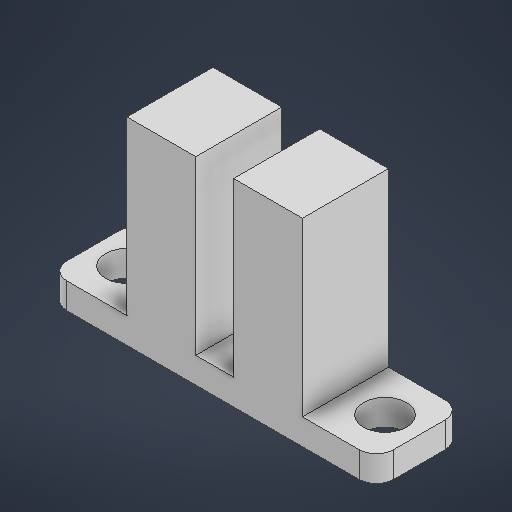
# Autodesk Inventor part: uchytka
Saved by Autodesk Inventor 2026.1 (Build 301233000, 233)
## iProperties
Created: 2026-01-08
Part Number: uchytka
Material: Všeobecné
Document SubType Name: Modeling
Designer: bubli
Density: 1 g/cm^3
Appearance: Výchozí
Author: bubli
Autodesk Inventor part; units mm, degrees
ref_plane "YZ Plane" through (0, 0, 0) normal (1, 0, 0) x (0, 1, 0)
ref_plane "XZ Plane" through (0, 0, 0) normal (0, 1, 0) x (-1, 0, 0)
ref_plane "XY Plane" through (0, 0, 0) normal (0, 0, 1) x (1, 0, 0)
sketch "Náčrt1" plane through (0, 0, 0) normal (0, 0, 1) x (1, 0, 0)
  line L0 (-6.3446, 3.6092) -> (27.6554, 3.6092)
  line L1 (29.6554, 1.6092) -> (29.6554, -4.3908)
  line L2 (27.6554, -6.3908) -> (-6.3446, -6.3908)
  line L3 (-8.3446, -4.3908) -> (-8.3446, 1.6092)
  circle A0 centre (-4.3446, -1.3908) radius 2.5
  circle A1 centre (25.6554, -1.3908) radius 2.5
  arc A2 (-6.3446, 3.6092) -> (-8.3446, 1.6092) centre (-6.3446, 1.6092) ccw
  arc A3 (29.6554, 1.6092) -> (27.6554, 3.6092) centre (27.6554, 1.6092) ccw
  arc A4 (27.6554, -6.3908) -> (29.6554, -4.3908) centre (27.6554, -4.3908) ccw
  arc A5 (-8.3446, -4.3908) -> (-6.3446, -6.3908) centre (-6.3446, -4.3908) ccw
  point P0 (0, 0)
  point P1 (-8.3446, 3.6092)
  point P2 (29.6554, 3.6092)
  point P3 (-8.3446, -6.3908)
  dimension "d0" = 38
  dimension "d1" = 10
  dimension "d2" = 5
  dimension "d3" = 5
  dimension "d4" = 5
  dimension "d5" = 5
  dimension "d6" = 4
  dimension "d7" = 4
  dimension "d8" = 2
  constraints: 8 end point, 8 point on circle, 8 tangent, 6 centre point, 6 point on line, 3 equal radius, 2 parallel, 1 horizontal, 1 perpendicular
  measures "d0" distance of point (-8.345, 3.609) point (29.655, 3.609)
  measures "d1" distance of point (-8.345, -6.391) point (-8.345, 3.609)
  measures "d2" diameter of A0
  measures "d3" diameter of A1
  measures "d4" distance from line of L0 A0.centre
  measures "d5" distance from line of L0 A1.centre
  measures "d6" distance from line of L3 A0.centre
  measures "d7" distance from line of L1 A1.centre
  measures "d8" radius of A2
extrude "Vysunutí1" add sketch "Náčrt1" along normal blind 3
sketch "Náčrt2" plane through (0, 0, 3) normal (0, 0, 1) x (1, 0, 0)
  line L0 (0.6554, 3.6092) -> (8.6554, 3.6092)
  line L1 (8.6554, 3.6092) -> (8.6554, -6.3908)
  line L2 (8.6554, -6.3908) -> (0.6554, -6.3908)
  line L3 (0.6554, -6.3908) -> (0.6554, 3.6092)
  line L4 (13.0554, 3.6092) -> (21.0554, 3.6092)
  line L5 (21.0554, 3.6092) -> (21.0554, -6.3908)
  line L6 (21.0554, -6.3908) -> (13.0554, -6.3908)
  line L7 (13.0554, -6.3908) -> (13.0554, 3.6092)
  line L8 (-8.3446, 1.6092) -> (-8.3446, -4.3908) projected
  line L9 (-6.3446, -6.3908) -> (27.6554, -6.3908) projected
  line L10 (27.6554, 3.6092) -> (-6.3446, 3.6092) projected
  point P0 (0, 0)
  point P1 (4.6554, -6.3908)
  dimension "d11" = 4.4
  dimension "d12" = 8
  dimension "d13" = 8
  dimension "d14" = 9
  dimension "d15" = 10
  dimension "d16" = 0
  dimension "d21" = 0
  constraints: 16 end point, 4 parallel, 2 horizontal, 2 perpendicular, 2 point on line, 1 midpoint
  measures "d11" distance between parallel lines of L7 L1
  measures "d12" distance between parallel lines of L5 L7
  measures "d13" distance of L0.start L0.end
  measures "d14" distance between parallel lines of L8 L3
  measures "d15" distance from line of point (4.655, -6.391) L0
  measures "d16" distance from line of L9 L2.end
  measures "d21" distance between parallel lines of L10 L0
extrude "Vysunutí2" add sketch "Náčrt2" along normal blind 20 contours L0 L1 L2 L3 | L4 L5 L6 L7
